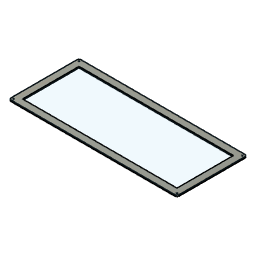
CapyBoard Top (Autodesk Fusion 360 design; units mm, degrees)
Autodesk Fusion 360 part; units mm, degrees
sketch "Sketch1" plane through (0, 0, 0) normal (0, 0, 1) x (1, 0, 0)
  line L0 (0, 0) -> (385.5, 0)
  line L1 (385.5, 0) -> (385.5, 160.5)
  line L2 (385.5, 160.5) -> (0, 160.5)
  line L3 (0, 160.5) -> (0, 0)
  line L4 (10, 150.5) -> (375.5, 150.5)
  line L5 (375.5, 150.5) -> (375.5, 10)
  line L6 (375.5, 10) -> (10, 10)
  line L7 (10, 10) -> (10, 150.5)
  circle A0 centre (5, 155.5) radius 1.45
  circle A1 centre (5, 5) radius 1.45
  circle A2 centre (380.5, 5) radius 1.45
  circle A3 centre (380.5, 155.5) radius 1.45
  dimension "d1" = 160.5
  dimension "d2" = 385.5
  dimension "d3" = 10
  dimension "d4" = 10
  dimension "d5" = 10
  dimension "d6" = 10
  dimension "d7" = 2.9
  dimension "d8" = 2.9
  dimension "d9" = 2.9
  dimension "d10" = 2.9
  dimension "d11" = 5
  dimension "d12" = 5
  dimension "d13" = 5
  dimension "d14" = 5
  dimension "d15" = 5
  dimension "d16" = 5
  dimension "d17" = 5
  dimension "d18" = 5
  constraint horizontal L0
  constraint vertical L1
  constraint horizontal L2
  constraint vertical L3
  constraint coincident L0.start L3.end
  constraint horizontal L4
  constraint vertical L5
  constraint horizontal L6
  constraint vertical L7
  measures "d1" distance of L0.start L2.end
  measures "d2" distance of L1 L3
  measures "d3" distance of L1 L5
  measures "d4" distance of L2 L4
  measures "d5" distance of L0 L6
  measures "d6" distance of L3 L7
  measures "d7" diameter of A0
  measures "d8" diameter of A1
  measures "d9" diameter of A2
  measures "d10" diameter of A3
  measures "d11" distance of L2 A3.centre
  measures "d12" distance of L1 A3.centre
  measures "d13" distance of L1 A2.centre
  measures "d14" distance of L0 A2.centre
  measures "d15" distance of L0 A1.centre
  measures "d16" distance of L3 A1.centre
  measures "d17" distance of L2 A0.centre
  measures "d18" distance of L3 A0.centre
sketch "Sketch2" plane through (0, 0, 0) normal (0, 0, 1) x (1, 0, 0)
  line L0 (0, 0) -> (385.5, 0)
  line L1 (385.5, 0) -> (385.5, 160.5)
  line L2 (385.5, 160.5) -> (0, 160.5)
  line L3 (0, 160.5) -> (0, 0)
  line L4 (375.5, 10) -> (10, 10)
  line L5 (10, 10) -> (10, 150.5)
  line L6 (10, 150.5) -> (375.5, 150.5)
  line L7 (375.5, 150.5) -> (375.5, 10)
  dimension "d21" = 160.5
  dimension "d22" = 385.5
  dimension "d23" = 10
  dimension "d24" = 10
  dimension "d25" = 365.5
  dimension "d26" = 140.5
  constraint horizontal L0
  constraint vertical L1
  constraint horizontal L2
  constraint vertical L3
  constraint coincident L0.start L3.end
  constraint horizontal L4
  constraint vertical L5
  constraint horizontal L6
  constraint vertical L7
  measures "d21" distance of L0.start L2.end
  measures "d22" distance of L1 L3
  measures "d23" distance of L3 L5
  measures "d24" distance of L0 L4
  measures "d25" distance of L5 L7
  measures "d26" distance of L4 L6
sketch "Sketch3" plane through (0, 0, 0) normal (0, 1, 0) x (1, 0, 0)
sketch "Sketch4" plane through (0, 0, 0) normal (0, 0, 1) x (1, 0, 0)
  line L0 (0, -20) -> (385.5, -20)
  line L1 (385.5, -20) -> (385.5, -180.5)
  line L2 (385.5, -180.5) -> (0, -180.5)
  line L3 (0, -180.5) -> (0, -20)
  line L4 (375.5, -170.5) -> (10, -170.5)
  line L5 (10, -170.5) -> (10, -30)
  line L6 (10, -30) -> (375.5, -30)
  line L7 (375.5, -30) -> (375.5, -170.5)
  circle A0 centre (5, -175.5) radius 1.45
  circle A1 centre (5, -25) radius 1.45
  circle A2 centre (380.5, -25) radius 1.45
  circle A3 centre (380.5, -175.5) radius 1.45
  dimension "d29" = 160.5
  dimension "d30" = 385.5
  dimension "d31" = 10
  dimension "d32" = 10
  dimension "d33" = 10
  dimension "d34" = 10
  dimension "d35" = 2.9
  dimension "d36" = 5
  dimension "d37" = 5
  dimension "d38" = 2.9
  dimension "d39" = 5
  dimension "d40" = 5
  dimension "d41" = 2.9
  dimension "d42" = 5
  dimension "d43" = 5
  dimension "d44" = 2.9
  dimension "d45" = 5
  dimension "d46" = 5
  constraint horizontal L0
  constraint vertical L1
  constraint horizontal L2
  constraint vertical L3
  constraint horizontal L4
  constraint vertical L5
  constraint horizontal L6
  constraint vertical L7
  measures "d29" distance of L0 L2
  measures "d30" distance of L1 L3
  measures "d31" distance of L3 L5
  measures "d32" distance of L1 L7
  measures "d33" distance of L2 L4
  measures "d34" distance of L0 L6
  measures "d35" diameter of A0
  measures "d36" distance of L2 A0.centre
  measures "d37" distance of L3 A0.centre
  measures "d38" diameter of A1
  measures "d39" distance of L0 A1.centre
  measures "d40" distance of L3 A1.centre
  measures "d41" diameter of A2
  measures "d42" distance of L0 A2.centre
  measures "d43" distance of L1 A2.centre
  measures "d44" diameter of A3
  measures "d45" distance of L2 A3.centre
  measures "d46" distance of L1 A3.centre
extrude "Extrude3" add sketch "Sketch4" along normal blind 3 contours L0 L1 L2 L3 | L4 L5 L6 L7
sketch "Sketch5" plane through (0, 0, 3) normal (0, 0, 1) x (-1, 0, 0)
  circle A0 centre (-15.5, -145) radius 3.3
  circle A1 centre (-15.5, -145) radius 1.3
  circle A2 centre (-15.5, -15.5) radius 1.3
  circle A3 centre (-15.5, -15.5) radius 3.3
  circle A4 centre (-370, -15.5) radius 1.3
  circle A5 centre (-370, -15.5) radius 3.3
  circle A6 centre (-370, -145) radius 1.3
  circle A7 centre (-370, -145) radius 3.3
  line L0 (-375.5, -150.5) -> (-10, -150.5)
  line L1 (-10, -150.5) -> (-10, -10)
  line L2 (-10, -10) -> (-375.5, -10)
  line L3 (-375.5, -10) -> (-375.5, -150.5)
  dimension "d49" = 6.6
  dimension "d52" = 2.6
  dimension "d53" = 2.6
  dimension "d56" = 6.6
  dimension "d57" = 2.6
  dimension "d58" = 6.6
  dimension "d61" = 2.6
  dimension "d62" = 6.6
  constraint concentric A0 A1
  constraint concentric A2 A3
  constraint concentric A4 A5
  constraint concentric A6 A7
  measures "d49" diameter of A0
  measures "d52" diameter of A1
  measures "d53" diameter of A2
  measures "d56" diameter of A3
  measures "d57" diameter of A4
  measures "d58" diameter of A5
  measures "d61" diameter of A6
  measures "d62" diameter of A7
sketch "Sketch6" plane through (0, 0, 3) normal (0, 0, 1) x (-1, 0, 0)
  circle A0 centre (-5, 25) radius 1.45
  circle A1 centre (-5, 175.5) radius 1.45
  circle A2 centre (-380.5, 25) radius 1.45
  circle A3 centre (-380.5, 175.5) radius 1.45
  line L0 (0, 180.5) -> (-385.5, 180.5)
  line L1 (-385.5, 180.5) -> (-385.5, 20)
  line L2 (-385.5, 20) -> (0, 20)
  line L3 (0, 20) -> (0, 180.5)
sketch "Sketch7" plane through (0, 0, 0) normal (0, 0, -1) x (1, 0, 0)
  circle A0 centre (5, 25) radius 1.45
  circle A1 centre (5, 175.5) radius 1.45
  circle A2 centre (380.5, 25) radius 1.45
  circle A3 centre (380.5, 175.5) radius 1.45
  line L0 (385.5, 180.5) -> (0, 180.5)
  line L1 (0, 180.5) -> (0, 20)
  line L2 (0, 20) -> (385.5, 20)
  line L3 (385.5, 20) -> (385.5, 180.5)
  line L4 (0, 20) -> (385.5, 20)
  line L5 (385.5, 20) -> (385.5, 180.5)
  line L6 (385.5, 180.5) -> (0, 180.5)
  line L7 (0, 180.5) -> (0, 20)
  line L8 (0, 20) -> (385.5, 20)
  line L9 (385.5, 20) -> (385.5, 180.5)
  line L10 (385.5, 180.5) -> (0, 180.5)
  line L11 (0, 180.5) -> (0, 20)
  line L12 (0, 20) -> (385.5, 20)
  line L13 (385.5, 20) -> (385.5, 180.5)
  line L14 (385.5, 180.5) -> (0, 180.5)
  line L15 (0, 180.5) -> (0, 20)
  line L16 (15.5, 165) -> (370, 165)
  line L17 (370, 165) -> (370, 35.5)
  line L18 (370, 35.5) -> (15.5, 35.5)
  line L19 (15.5, 35.5) -> (15.5, 165)
  line L20 (0, 180.5) -> (385.5, 180.5)
  dimension "d68" = 15.5
  dimension "d70" = 15.5
  dimension "d71" = 15.5
  dimension "d72" = 15.5
  constraint horizontal L4
  constraint vertical L5
  constraint horizontal L6
  constraint vertical L7
  constraint coincident L0.start L3.end
  constraint coincident L1.end L2.start
  constraint horizontal L8
  constraint vertical L9
  constraint horizontal L10
  constraint vertical L11
  constraint horizontal L12
  constraint vertical L13
  constraint horizontal L14
  constraint vertical L15
  constraint horizontal L16
  constraint vertical L17
  constraint horizontal L18
  constraint vertical L19
  measures "d68" distance of L13 L17
  measures "d70" distance of L7 L19
  measures "d71" distance of L16 L20
  measures "d72" distance of L4 L18
extrude "Extrude5" cut sketch "Sketch7" against normal blind 150 contours L16 L17 L18 L19
fillet "Fillet5" radius 4 1 edges at (385.5, -180.5, 1.5)
fillet "Fillet6" radius 4 1 edges at (385.5, -20, 1.5)
fillet "Fillet7" radius 4 1 edges at (0, -180.5, 1.5)
fillet "Fillet8" radius 4 1 edges at (0, -20, 1.5)
